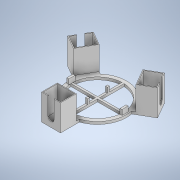
# Autodesk Inventor part: bottom
Saved by Autodesk Inventor 2020 (Build 240168000, 168)
## iProperties
Created: 2020-03-22
Part Number: bottom
Material: Generic
Document SubType Name: Modeling
Designer: Tarsoly
Density: 1 g/cm^3
Appearance: Default
Author: Tarsoly
Autodesk Inventor part; units mm, degrees
ref_plane "YZ Plane" through (0, 0, 0) normal (1, 0, 0) x (0, 1, 0)
ref_plane "XZ Plane" through (0, 0, 0) normal (0, 1, 0) x (-1, 0, 0)
ref_plane "XY Plane" through (0, 0, 0) normal (0, 0, 1) x (1, 0, 0)
sketch "Sketch1" plane through (0, 0, 0) normal (0, 1, 0) x (-1, 0, 0)
  circle A0 centre (0, 0) radius 57
  circle A1 centre (0, 0) radius 50
  line L0 (0, -92.0258) -> (0, 121.5043) projected
  line L1 (123.2816, 0) -> (-123.2816, 0) projected
  line L2 (-50, 2) -> (50, 2)
  line L3 (50, 2) -> (50, -2)
  line L4 (50, -2) -> (-50, -2)
  line L5 (-50, -2) -> (-50, 2)
  line L6 (-50, 2) -> (50, -2) construction
  line L7 (50, 2) -> (-50, -2) construction
  line L8 (2, 50) -> (-2, 50)
  line L9 (-2, 50) -> (-2, -50)
  line L10 (-2, -50) -> (2, -50)
  line L11 (2, -50) -> (2, 50)
  line L12 (2, 50) -> (-2, -50) construction
  line L13 (-2, 50) -> (2, -50) construction
  line L14 (18.5, 91) -> (-18.5, 91)
  line L15 (-18.5, 91) -> (-18.5, 50)
  line L16 (-18.5, 50) -> (18.5, 50)
  line L17 (18.5, 50) -> (18.5, 91)
  line L18 (0, 91) -> (0, 50) construction
  line L19 (18.5, 60) -> (-18.5, 60)
  line L20 (-44.3013, -23.2679) -> (-42.3013, -26.7321)
  line L21 (-34.0513, -41.0215) -> (-52.5513, -8.9785)
  line L22 (-61.2115, -13.9785) -> (-42.7115, -46.0215)
  line L23 (-69.5583, -61.5215) -> (-34.0513, -41.0215)
  line L24 (-52.5513, -8.9785) -> (-88.0583, -29.4785)
  line L25 (-78.8083, -45.5) -> (-43.3013, -25) construction
  line L26 (-88.0583, -29.4785) -> (-69.5583, -61.5215)
  line L27 (42.3013, -26.7321) -> (44.3013, -23.2679)
  line L28 (52.5513, -8.9785) -> (34.0513, -41.0215)
  line L29 (42.7115, -46.0215) -> (61.2115, -13.9785)
  line L30 (88.0583, -29.4785) -> (52.5513, -8.9785)
  line L31 (34.0513, -41.0215) -> (69.5583, -61.5215)
  line L32 (78.8083, -45.5) -> (43.3013, -25) construction
  line L33 (69.5583, -61.5215) -> (88.0583, -29.4785)
  point P0 (2, -49.96)
  point P1 (2, -2)
  point P2 (49.96, -2)
  point P3 (-2, 49.96)
  point P4 (-2, 2)
  point P5 (-49.96, 2)
  point P6 (-2, -49.96)
  point P7 (-49.96, -2)
  point P8 (-2, -2)
  point P9 (-18.5, 53.9143)
  point P10 (-55.9411, -10.9357)
  point P11 (-37.4411, -42.9786)
  point P12 (37.4411, -42.9786)
  point P13 (55.9411, -10.9357)
  point P14 (18.5, 53.9143)
  point P15 (2, 49.96)
  point P16 (49.96, 2)
  point P17 (2, 2)
  dimension "d0" = 114
  dimension "d1" = 100
  dimension "d6" = 100
  dimension "d7" = 4
  dimension "d8" = 4
  dimension "d9" = 100
  dimension "d10" = 37
  dimension "d14" = 60
  dimension "d15" = 31
  dimension "d18" = 360
  constraints: 64 end point, 6 midpoint, 6 parallel, 6 point on line, 4 perpendicular, 3 horizontal, 2 centre point, 2 coincident, 1 collinear, 1 tangent, 52 other
  measures "d0" diameter of A0
  measures "d1" diameter of A1
  measures "d6" distance of L3.end L4.end
  measures "d7" distance of L2.end L3.end
  measures "d8" distance of L10.end L9.end
  measures "d9" distance of L9.end L8.end
  measures "d10" distance of L16.end L15.end
  measures "d14" distance between parallel lines of L1 L19
  measures "d15" distance between parallel lines of L19 L14
extrude "Extrusion1" add sketch "Sketch1" along normal blind 5 contours L1 L3 L2 A1 L11 L16 L17 A0 | A0 L30 L28 L27 A1 L4 L3 L1 | L17 L16 L8 L0 A0 | A0 L0 L19 L17 | L30 L29 L31 A0 | A0 L31 L28 L27 L30 | L1 L11 L2 A1 | L3 L4 A1 | A1 L4 L11 L1 | A1 L2 L3 | L0 L8 L16 L15 A0 | A0 L15 L19 L0 | L19 L0 L14 L17 | A0 L0 L10 L11 A1 L27 L28 L31 | L30 L33 L31 L29 | L11 L4 L0 L1 | L1 L0 L2 L11 | L15 L16 L9 A1 L2 L5 L1 A0 | L8 L11 A1 | L0 L2 L9 A1 | A1 L11 L2 L0 | A1 L9 L8 | L19 L15 L14 L0 | A0 L23 L21 L20 A1 L9 L10 L0 | L11 A1 L0 L4 | L1 L9 L2 L0 | L0 L4 L9 L1 | L1 L5 L4 A1 L20 L21 L24 A0 | L23 L22 L24 A0 | A0 L24 L21 L20 L23 | L10 L9 A1 | A1 L9 L4 L0 | A1 L11 L10 | L9 L4 A1 L1 | L1 A1 L2 L9 | L5 L2 A1 | A1 L4 L5 | L23 L26 L24 L22
sketch "Sketch2" plane through (0, 5, 0) normal (0, 1, 0) x (1, 0, 0)
  line L0 (-18.5, -53.9143) -> (-18.5, -91) projected
  line L1 (18.5, -91) -> (18.5, -53.9143) projected
  line L2 (-18.5, -91) -> (18.5, -91)
  line L3 (18.5, -91) -> (18.5, -60)
  line L4 (18.5, -60) -> (-18.5, -60)
  line L5 (-18.5, -60) -> (-18.5, -91)
  line L6 (-17, -61.5) -> (17, -61.5)
  line L7 (17, -61.5) -> (17, -89.5)
  line L8 (17, -89.5) -> (-17, -89.5)
  line L9 (-17, -89.5) -> (-17, -61.5)
  line L10 (88.0583, 29.4785) -> (69.5583, 61.5215)
  line L11 (69.5583, 61.5215) -> (42.7115, 46.0215)
  line L12 (42.7115, 46.0215) -> (61.2115, 13.9785)
  line L13 (61.2115, 13.9785) -> (88.0583, 29.4785)
  line L14 (61.7606, 16.0276) -> (44.7606, 45.4724)
  line L15 (44.7606, 45.4724) -> (69.0093, 59.4724)
  line L16 (69.0093, 59.4724) -> (86.0093, 30.0276)
  line L17 (86.0093, 30.0276) -> (61.7606, 16.0276)
  line L18 (-69.5583, 61.5215) -> (-88.0583, 29.4785)
  line L19 (-88.0583, 29.4785) -> (-61.2115, 13.9785)
  line L20 (-61.2115, 13.9785) -> (-42.7115, 46.0215)
  line L21 (-42.7115, 46.0215) -> (-69.5583, 61.5215)
  line L22 (-44.7606, 45.4724) -> (-61.7606, 16.0276)
  line L23 (-61.7606, 16.0276) -> (-86.0093, 30.0276)
  line L24 (-86.0093, 30.0276) -> (-69.0093, 59.4724)
  line L25 (-69.0093, 59.4724) -> (-44.7606, 45.4724)
  point P0 (0, 0)
  dimension "d22" = 31
  dimension "d23" = 1.5
  dimension "d26" = 360
  constraints: 48 end point, 4 parallel, 2 perpendicular, 1 horizontal, 1 point on line, 52 other
  measures "d22" distance between parallel lines of L4 L2
  measures "d23" distance between parallel lines of L4 L6
extrude "Extrusion2" add sketch "Sketch2" along normal blind 46 contours L4 L1 L2 L0
sketch "Sketch4" plane through (-18.5, 0, 91) normal (0, 0, 1) x (1, 0, 0)
  line L0 (0, 51) -> (37, 51) construction
  line L1 (12.5, 51) -> (24.5, 51)
  line L2 (24.5, 51) -> (24.5, 10)
  line L3 (24.5, 10) -> (12.5, 10)
  line L4 (12.5, 10) -> (12.5, 51)
  line L5 (1.5, 5) -> (35.5, 5) construction
  line L6 (18.5, -10.2) -> (18.5, 61.2) construction
  circle A0 centre (18.5, 16) radius 6
  point P0 (18.5, 0)
  point P1 (12.5, 16)
  point P2 (24.5, 16)
  dimension "d36" = 12
  dimension "d37" = 5
  dimension "d38" = 6
  constraints: 8 end point, 2 parallel, 2 point on line, 2 tangent, 1 centre point, 1 horizontal, 1 perpendicular
  measures "d36" distance of L2.end L3.end
  measures "d37" distance between parallel lines of L5 L3
  measures "d38" distance between parallel lines of L6 L4
extrude "Extrusion3" cut sketch "Sketch4" against normal up to next contours L1 L2 A0 L4 | A0
pattern_circular "Circular Pattern1" count 3 over 360 about axis through (0, -10, 0) along (0, 1, 0) of "Extrusion2", "Extrusion3"
sketch "Sketch5" plane through (0, 5, 0) normal (0, 1, 0) x (1, 0, 0)
  line L0 (-2, -21.5) -> (2, -21.5)
  line L1 (2, -21.5) -> (2, -17.5)
  line L2 (2, -17.5) -> (-2, -17.5)
  line L3 (-2, -17.5) -> (-2, -21.5)
  line L4 (-2, -2) -> (-2, -49.96) construction
  line L5 (2, -49.96) -> (2, -2) construction
  line L6 (-123.2816, 0) -> (123.2816, 0) construction
  line L7 (-2, 21.5) -> (2, 21.5)
  line L8 (2, 21.5) -> (2, 17.5)
  line L9 (2, 17.5) -> (-2, 17.5)
  line L10 (-2, 17.5) -> (-2, 21.5)
  arc A0 (-49.96, -2) -> (-2, -49.96) centre (0, 0) ccw construction
  arc A1 (-2, 49.96) -> (-49.96, 2) centre (0, 0) ccw construction
  circle A2 centre (0, 0) radius 50 construction
  line L11 (-54, 6) -> (-50, 6)
  line L12 (-50, 6) -> (-50, -6)
  line L13 (-50, -6) -> (-54, -6)
  line L14 (-54, -6) -> (-54, 6)
  line L15 (-54, 0) -> (-50, 0) construction
  line L16 (0, 92.0258) -> (0, -121.5043) construction
  line L17 (54, 6) -> (50, 6)
  line L18 (50, 6) -> (50, -6)
  line L19 (50, -6) -> (54, -6)
  line L20 (54, -6) -> (54, 6)
  line L21 (54, 0) -> (50, 0) construction
  point P0 (49.96, -2)
  point P1 (49.96, 2)
  dimension "d41" = 17.5
  dimension "d42" = 4
  dimension "d43" = 12
  constraints: 36 end point, 12 symmetric about line, 4 parallel, 3 collinear, 3 perpendicular, 2 horizontal, 2 midpoint, 1 centre point, 1 coincident, 1 concentric, 1 tangent
  measures "d41" distance from line of point (0, 0) L2
  measures "d42" distance of L12.end L13.end
  measures "d43" distance of L11.end L12.end
extrude "Extrusion4" add sketch "Sketch5" along normal blind 10
equation "\"d38\" = 0.5 * d36"
body "Solid1"
